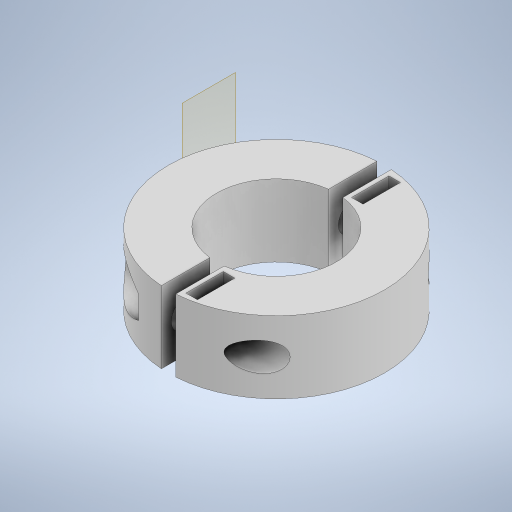
# Autodesk Inventor part: collar
Saved by Autodesk Inventor 2023 (Build 270158000, 158)
## iProperties
Created: 2022-11-03
Part Number: collar
Material: Generic
Document SubType Name: Modeling
Designer: neera
Density: 1 g/cm^3
Appearance: Default
Author: neera
Autodesk Inventor part; units mm, degrees
ref_plane "YZ Plane" through (0, 0, 0) normal (1, 0, 0) x (0, 1, 0)
ref_plane "XZ Plane" through (0, 0, 0) normal (0, 1, 0) x (-1, 0, 0)
ref_plane "XY Plane" through (0, 0, 0) normal (0, 0, 1) x (1, 0, 0)
sketch "Sketch1" plane through (0, 0, 0) normal (0, 1, 0) x (-1, 0, 0)
  circle A0 centre (0, 0) radius 4.15
  circle A1 centre (0, 0) radius 7.5
  dimension "d0" = 8.3
  dimension "d1" = 15
  constraints: 2 centre point, 2 coincident
  measures "d0" diameter of A0
  measures "d1" diameter of A1
extrude "Extrusion1" add sketch "Sketch1" along normal blind 5
sketch "Sketch2" plane through (0, 5, 0) normal (0, 1, 0) x (1, 0, 0)
  line L0 (-0.5, -8.297) -> (0.5, -8.297)
  line L1 (0.5, -8.297) -> (0.5, 8.8641)
  line L2 (0.5, 8.8641) -> (-0.5, 8.8641)
  line L3 (-0.5, 8.8641) -> (-0.5, -8.297)
  point P0 (0, 0)
  dimension "d4" = 1
  dimension "d5" = 0.5
  constraints: 8 end point, 2 parallel, 1 horizontal, 1 perpendicular
  measures "d4" distance of L2.end L1.end
  measures "d5" distance from line of point (0, 0) L3
extrude "Extrusion2" cut sketch "Sketch2" against normal blind 5
sketch "Sketch3" plane through (-0.5, 5, -4.1198) normal (1, 0, 0) x (0, 0, -1)
  circle A0 centre (1.6815, -2.5) radius 1
  line L0 (3.3635, -5) -> (3.3635, 0) projected
  line L1 (3.3635, -5) -> (-11.6031, -5) projected
  circle A1 centre (-9.9211, -2.5) radius 1
  line L2 (3.3635, 0) -> (-11.6031, 0) projected
  line L3 (-11.6031, 0) -> (-11.6031, -5) projected
  point P0 (-4.1198, -5)
  dimension "d8" = 2
  dimension "d9" = 1.682
  dimension "d10" = 2.5
  dimension "d11" = 2
  dimension "d12" = 2.5
  dimension "d13" = 1.682
  constraints: 2 centre point
  measures "d8" diameter of A0
  measures "d9" distance from line of L0 A0.centre
  measures "d10" distance from line of A0.centre L1
  measures "d11" diameter of A1
  measures "d12" distance from line of L2 A1.centre
  measures "d13" distance from line of L3 A1.centre
extrude "Extrusion3" cut sketch "Sketch3" along normal mid plane 20 contours A0 | A1
ref_plane "Work Plane1" through (-10.5, 5, -4.1198) normal (1, 0, 0) x (0, 0, -1)
sketch "Sketch4" plane through (-10.5, 5, -4.1198) normal (1, 0, 0) x (0, 0, -1)
  circle A0 centre (1.6815, -2.5) radius 1.5
  circle A1 centre (-9.9211, -2.5) radius 1.5
  circle A2 centre (-9.9211, -2.5) radius 1 projected
  circle A3 centre (1.6815, -2.5) radius 1 projected
  point P0 (-4.1198, -5)
  dimension "d17" = 3
  dimension "d18" = 3
  constraints: 2 centre point, 2 concentric
  measures "d17" diameter of A0
  measures "d18" diameter of A1
extrude "Extrusion4" cut sketch "Sketch4" along normal blind 8 contours A0 | A1 | A2 | A3
sketch "Sketch5" plane through (0, 5, 0) normal (0, 1, 0) x (1, 0, 0)
  line L0 (0.8, -7.0833) -> (1.6, -7.0833)
  line L1 (1.6, -7.0833) -> (1.6, -4.4833)
  line L2 (1.6, -4.4833) -> (0.8, -4.4833)
  line L3 (0.8, -4.4833) -> (0.8, -7.0833)
  line L4 (0.8, 4.4167) -> (1.6, 4.4167)
  line L5 (1.6, 4.4167) -> (1.6, 7.0167)
  line L6 (1.6, 7.0167) -> (0.8, 7.0167)
  line L7 (0.8, 7.0167) -> (0.8, 4.4167)
  line L8 (0.5, -4.1198) -> (0.5, -7.4833) projected
  point P0 (0, 0)
  point P1 (0.5, -5.8015)
  point P2 (1.2, -7.0833)
  point P3 (1.2, 4.4167)
  point P4 (1.2, -4.4833)
  dimension "d21" = 0.8
  dimension "d22" = 2.6
  dimension "d23" = 0.8
  dimension "d24" = 0.3
  dimension "d25" = 0.4
  dimension "d26" = 8.9
  dimension "d27" = 2.6
  constraints: 16 end point, 4 midpoint, 4 parallel, 2 horizontal, 2 perpendicular, 1 point on line
  measures "d21" distance of L6.end L5.end
  measures "d22" distance of L5.end L4.end
  measures "d23" distance between parallel lines of L1 L3
  measures "d24" distance from line of point (0.5, -5.802) L3
  measures "d25" vertical distance of L8.end point (1.2, -7.083)
  measures "d26" distance of point (1.2, 4.417) point (1.2, -4.483)
  measures "d27" distance of L0.end L1.end
extrude "Extrusion5" cut sketch "Sketch5" against normal blind 8
body "Solid1"
